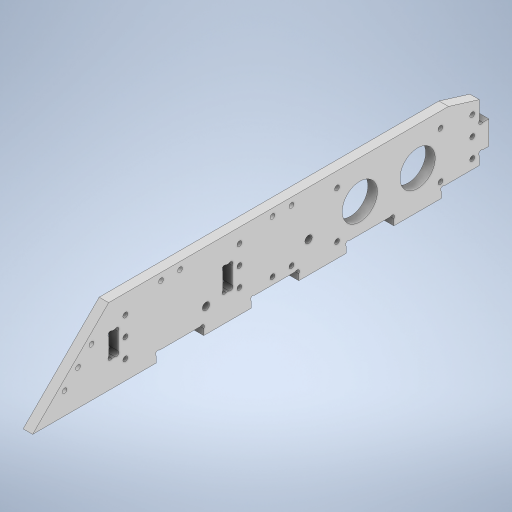
# Autodesk Inventor part: Inner Side Wall
Saved by Autodesk Inventor 2023 (Build 270158000, 158)
## iProperties
Created: 2022-12-26
Part Number: Inner Side Wall
Material: Generic
Document SubType Name: Modeling
Designer: justi
Density: 1 g/cm^3
Appearance: Default
Mass: 603.336 g
Surface Area: 1244.42 cm^2
Volume: 603.336 cm^3
Author: justi
Autodesk Inventor part; units mm, degrees
ref_plane "YZ Plane" through (0, 0, 0) normal (1, 0, 0) x (0, 1, 0)
ref_plane "XZ Plane" through (0, 0, 0) normal (0, 1, 0) x (-1, 0, 0)
ref_plane "XY Plane" through (0, 0, 0) normal (0, 0, 1) x (1, 0, 0)
sketch "Sketch1" plane through (0, 0, 0) normal (1, 0, 0) x (0, 1, 0)
  line L0 (0, 0) -> (101.6, 0)
  line L1 (101.6, 0) -> (101.6, -508)
  line L2 (101.6, -508) -> (0, -508)
  line L3 (0, -508) -> (0, 0)
  line L4 (0, 0) -> (0, 101.6)
  line L5 (0, 101.6) -> (101.6, 0)
  circle A0 centre (50.8, -412.75) radius 20.6375
  circle A1 centre (81.788, -443.23) radius 3.175
  circle A2 centre (19.812, -443.23) radius 3.175
  circle A3 centre (81.788, -305.054) radius 3.175
  circle A4 centre (19.812, -305.054) radius 3.175
  line L6 (66.675, 0) -> (34.925, 0)
  line L7 (34.925, 0) -> (34.925, -12.7)
  line L8 (34.925, -12.7) -> (66.675, -12.7)
  line L9 (66.675, -12.7) -> (66.675, 0)
  line L10 (66.675, -152.4) -> (34.925, -152.4)
  line L11 (34.925, -152.4) -> (34.925, -165.1)
  line L12 (34.925, -165.1) -> (66.675, -165.1)
  line L13 (66.675, -165.1) -> (66.675, -152.4)
  line L14 (0, -63.5) -> (12.7, -63.5)
  line L15 (12.7, -63.5) -> (12.7, -127)
  line L16 (12.7, -127) -> (0, -127)
  line L17 (0, -127) -> (0, -63.5)
  line L18 (0, -190.5) -> (12.7, -190.5)
  line L19 (12.7, -190.5) -> (12.7, -254)
  line L20 (12.7, -254) -> (0, -254)
  line L21 (0, -254) -> (0, -190.5)
  line L22 (0, -317.5) -> (12.7, -317.5)
  line L23 (12.7, -317.5) -> (12.7, -381)
  line L24 (12.7, -381) -> (0, -381)
  line L25 (0, -381) -> (0, -317.5)
  line L26 (0, -444.5) -> (12.7, -444.5)
  line L27 (12.7, -444.5) -> (12.7, -508)
  line L28 (12.7, -508) -> (0, -508)
  line L29 (0, -508) -> (0, -444.5)
  point P0 (0, -127)
  point P1 (0, -254)
  point P2 (0, -381)
  dimension "d0" = 508
  dimension "d1" = 101.6
  dimension "d2" = 101.6
  dimension "d3" = 41.275
  dimension "d4" = 50.8
  dimension "d5" = 95.25
  dimension "d6" = 6.35
  dimension "d7" = 30.48
  dimension "d8" = 30.988
  dimension "d9" = 6.35
  dimension "d10" = 30.48
  dimension "d11" = 30.988
  dimension "d12" = 6.35
  dimension "d13" = 107.696
  dimension "d14" = 6.35
  dimension "d15" = 107.696
  dimension "d16" = 30.988
  dimension "d17" = 30.988
  dimension "d18" = 31.75
  dimension "d19" = 12.7
  dimension "d20" = 34.925
  dimension "d21" = 31.75
  dimension "d22" = 34.925
  dimension "d23" = 139.7
  dimension "d24" = 12.7
  dimension "d25" = 12.7
  dimension "d26" = 63.5
  dimension "d27" = 63.5
  dimension "d28" = 12.7
  dimension "d29" = 63.5
  dimension "d30" = 63.5
  dimension "d31" = 12.7
  dimension "d32" = 63.5
  dimension "d33" = 63.5
  dimension "d34" = 12.7
  dimension "d35" = 63.5
  dimension "d36" = 63.5
  constraints: 60 end point, 14 parallel, 7 horizontal, 7 perpendicular, 5 centre point, 5 point on line, 1 vertical
  measures "d0" distance of L0.end L1.end
  measures "d1" distance of L1.end L2.end
  measures "d2" distance of L0.start L4.end
  measures "d3" diameter of A0
  measures "d4" distance from line of L1 A0.centre
  measures "d5" distance from line of L2 A0.centre
  measures "d6" diameter of A1
  measures "d7" vertical distance of A0.centre A1.centre
  measures "d8" horizontal distance of A0.centre A1.centre
  measures "d9" diameter of A2
  measures "d10" vertical distance of A0.centre A2.centre
  measures "d11" horizontal distance of A0.centre A2.centre
  measures "d12" diameter of A3
  measures "d13" vertical distance of A0.centre A3.centre
  measures "d14" diameter of A4
  measures "d15" vertical distance of A0.centre A4.centre
  measures "d16" horizontal distance of A4.centre A0.centre
  measures "d17" horizontal distance of A3.centre A0.centre
  measures "d18" distance of L8.end L7.end
  measures "d19" distance of L8.end L6.start
  measures "d20" distance between parallel lines of L1 L9
  measures "d21" distance of L12.end L11.end
  measures "d22" distance between parallel lines of L1 L13
  measures "d23" distance between parallel lines of L8 L10
  measures "d24" distance of L10.end L11.end
  measures "d25" distance of L15.end L16.end
  measures "d26" distance of L14.end L15.end
  measures "d27" distance between parallel lines of L0 L14
  measures "d28" distance of L19.end L20.end
  measures "d29" distance of L18.end L19.end
  measures "d30" distance between parallel lines of L16 L18
  measures "d31" distance of L23.end L24.end
  measures "d32" distance of L22.end L23.end
  measures "d33" distance between parallel lines of L20 L22
  measures "d34" distance of L27.end L28.end
  measures "d35" distance of L26.end L27.end
  measures "d36" distance between parallel lines of L24 L26
extrude "Extrusion1" add sketch "Sketch1" along normal blind 12.7 contours L4 L5 L0 | L0 L7 L8 L9 L1 L2 L27 L26 L3 L24 L23 L22 L20 L19 L18 L16 L15 L14
sketch "Sketch4" plane through (12.7, 0, 0) normal (1, 0, 0) x (0, 0, -1)
  line L0 (444.5, 12.7) -> (508, 12.7) projected
  line L1 (508, 12.7) -> (495.3, 12.7)
  line L2 (495.3, 12.7) -> (495.3, 28.575)
  line L3 (495.3, 28.575) -> (508, 28.575)
  line L4 (508, 28.575) -> (508, 12.7)
  line L5 (508, 101.6) -> (0, 101.6) projected
  line L6 (508, 101.6) -> (495.3, 101.6)
  line L7 (495.3, 101.6) -> (495.3, 60.325)
  line L8 (495.3, 60.325) -> (508, 60.325)
  line L9 (508, 60.325) -> (508, 101.6)
  circle A0 centre (412.75, 50.8) radius 20.6375 projected
  line L10 (412.75, 50.8) -> (400.05, 50.8)
  line L11 (400.05, 50.8) -> (400.05, 114.3)
  line L12 (400.05, 114.3) -> (412.75, 114.3)
  line L13 (412.75, 114.3) -> (412.75, 50.8)
  line L14 (412.75, 114.3) -> (495.3, 88.9)
  line L15 (495.3, 101.6) -> (495.3, 88.9)
  line L16 (495.3, 101.6) -> (454.025, 101.6)
  point P0 (0, 0)
  dimension "d39" = 12.7
  dimension "d40" = 15.875
  dimension "d41" = 12.7
  dimension "d42" = 31.75
  dimension "d43" = 12.7
  dimension "d44" = 63.5
  dimension "d45" = 12.7
  constraints: 30 end point, 6 parallel, 3 horizontal, 3 perpendicular, 2 point on line, 1 collinear, 1 midpoint
  measures "d39" distance of L2.end L3.end
  measures "d40" distance of L1.end L2.end
  measures "d41" distance of L8.end L7.end
  measures "d42" distance between parallel lines of L3 L8
  measures "d43" distance of L11.end L12.end
  measures "d44" distance of L12.end L10.start
  measures "d45" distance of L6.end L14.end
extrude "Extrusion2" cut sketch "Sketch4" against normal blind 12.7 contours L2 L3 L4 L0 | L9 L8 L7 L5 | L7 L14 L5
sketch "Sketch10" plane through (12.7, 0, 0) normal (1, 0, 0) x (0, 0, -1)
  line L0 (0, 66.675) -> (2.2451, 64.4299)
  line L1 (0, 66.675) -> (12.7, 66.675) projected
  line L2 (12.7, 66.675) -> (10.4549, 64.4299)
  line L3 (12.7, 66.675) -> (12.7, 34.925) projected
  line L4 (12.7, 34.925) -> (0, 34.925) projected
  line L5 (0, 34.925) -> (2.2451, 37.1701)
  line L6 (12.7, 34.925) -> (10.4549, 37.1701)
  line L7 (63.5, 12.7) -> (65.7451, 10.4549)
  line L8 (63.5, 12.7) -> (127, 12.7) projected
  line L9 (127, 12.7) -> (127, 0) projected
  line L10 (127, 12.7) -> (124.7549, 10.4549)
  line L11 (152.4, 34.925) -> (152.4, 66.675) projected
  line L12 (152.4, 66.675) -> (154.6451, 64.4299)
  line L13 (152.4, 66.675) -> (165.1, 66.675) projected
  line L14 (165.1, 66.675) -> (165.1, 34.925) projected
  line L15 (165.1, 66.675) -> (162.8549, 64.4299)
  line L16 (165.1, 34.925) -> (152.4, 34.925) projected
  line L17 (152.4, 34.925) -> (154.6451, 37.1701)
  line L18 (165.1, 34.925) -> (162.8549, 37.1701)
  line L19 (190.5, 0) -> (190.5, 12.7) projected
  line L20 (190.5, 12.7) -> (192.7451, 10.4549)
  line L21 (190.5, 12.7) -> (254, 12.7) projected
  line L22 (254, 12.7) -> (251.7549, 10.4549)
  line L23 (254, 12.7) -> (254, 0) projected
  line L24 (317.5, 0) -> (317.5, 12.7) projected
  line L25 (317.5, 12.7) -> (319.7451, 10.4549)
  line L26 (317.5, 12.7) -> (381, 12.7) projected
  line L27 (381, 12.7) -> (381, 0) projected
  line L28 (381, 12.7) -> (378.7549, 10.4549)
  line L29 (444.5, 0) -> (444.5, 12.7) projected
  line L30 (444.5, 12.7) -> (446.7451, 10.4549)
  line L31 (444.5, 12.7) -> (495.3, 12.7) projected
  line L32 (495.3, 12.7) -> (495.3, 28.575) projected
  line L33 (495.3, 28.575) -> (497.5451, 26.3299)
  line L34 (495.3, 28.575) -> (508, 28.575) projected
  line L35 (495.3, 60.325) -> (508, 60.325) projected
  line L36 (495.3, 60.325) -> (497.5451, 62.5701)
  circle A0 centre (497.5451, 62.5701) radius 3.175
  circle A1 centre (497.5451, 26.3299) radius 3.175
  circle A2 centre (446.7451, 10.4549) radius 3.175
  circle A3 centre (378.7549, 10.4549) radius 3.175
  circle A4 centre (319.7451, 10.4549) radius 3.175
  circle A5 centre (251.7549, 10.4549) radius 3.175
  circle A6 centre (192.7451, 10.4549) radius 3.175
  circle A7 centre (154.6451, 64.4299) radius 3.175
  circle A8 centre (162.8549, 64.4299) radius 3.175
  circle A9 centre (154.6451, 37.1701) radius 3.175
  circle A10 centre (162.8549, 37.1701) radius 3.175
  circle A11 centre (2.2451, 37.1701) radius 3.175
  circle A12 centre (10.4549, 37.1701) radius 3.175
  circle A13 centre (2.2451, 64.4299) radius 3.175
  circle A14 centre (10.4549, 64.4299) radius 3.175
  circle A15 centre (65.7451, 10.4549) radius 3.175
  circle A16 centre (124.7549, 10.4549) radius 3.175
  point P0 (0, 0)
  dimension "d53" = 3.175
  dimension "d54" = 45
  dimension "d55" = 3.175
  dimension "d56" = 45
  dimension "d57" = 3.175
  dimension "d58" = 45
  dimension "d59" = 3.175
  dimension "d60" = 45
  dimension "d61" = 3.175
  dimension "d62" = 45
  dimension "d63" = 3.175
  dimension "d64" = 45
  dimension "d65" = 3.175
  dimension "d66" = 45
  dimension "d67" = 3.175
  dimension "d68" = 45
  dimension "d69" = 3.175
  dimension "d70" = 45
  dimension "d71" = 3.175
  dimension "d72" = 45
  dimension "d73" = 3.175
  dimension "d74" = 45
  dimension "d75" = 3.175
  dimension "d76" = 45
  dimension "d77" = 3.175
  dimension "d78" = 45
  dimension "d79" = 3.175
  dimension "d80" = 45
  dimension "d81" = 3.175
  dimension "d82" = 45
  dimension "d83" = 3.175
  dimension "d84" = 45
  dimension "d85" = 3.175
  dimension "d86" = 45
  dimension "d87" = 6.35
  dimension "d88" = 6.35
  dimension "d89" = 6.35
  dimension "d90" = 6.35
  dimension "d91" = 6.35
  dimension "d92" = 6.35
  dimension "d93" = 6.35
  dimension "d94" = 6.35
  dimension "d95" = 6.35
  dimension "d96" = 6.35
  dimension "d97" = 6.35
  dimension "d98" = 6.35
  dimension "d99" = 6.35
  dimension "d100" = 6.35
  dimension "d101" = 6.35
  dimension "d102" = 6.35
  dimension "d103" = 6.35
  constraints: 34 end point, 17 centre point, 12 point on line
  measures "d53" distance of L0.start L0.end
  measures "d54" angle of L1 L0
  measures "d55" distance of L1.end L2.end
  measures "d56" angle of L3 L2
  measures "d57" distance of L4.end L5.end
  measures "d58" angle of L4 L5
  measures "d59" distance of L3.end L6.end
  measures "d60" angle of L3 L6
  measures "d61" distance of L7.start L7.end
  measures "d62" angle of L8 L7
  measures "d63" distance of L8.end L10.end
  measures "d64" angle of L9 L10
  measures "d65" distance of L11.end L12.end
  measures "d66" angle of L13 L12
  measures "d67" distance of L13.end L15.end
  measures "d68" angle of L14 L15
  measures "d69" distance of L11.start L17.end
  measures "d70" angle of L16 L17
  measures "d71" distance of L14.end L18.end
  measures "d72" angle of L14 L18
  measures "d73" distance of L19.end L20.end
  measures "d74" angle of L21 L20
  measures "d75" distance of L21.end L22.end
  measures "d76" angle of L23 L22
  measures "d77" distance of L24.end L25.end
  measures "d78" angle of L26 L25
  measures "d79" distance of L26.end L28.end
  measures "d80" angle of L27 L28
  measures "d81" distance of L29.end L30.end
  measures "d82" angle of L31 L30
  measures "d83" distance of L32.end L33.end
  measures "d84" angle of L34 L33
  measures "d85" distance of L35.start L36.end
  measures "d86" angle of L35 L36
  measures "d87" diameter of A0
  measures "d88" diameter of A1
  measures "d89" diameter of A2
  measures "d90" diameter of A3
  measures "d91" diameter of A4
  measures "d92" diameter of A5
  measures "d93" diameter of A6
  measures "d94" diameter of A7
  measures "d95" diameter of A8
  measures "d96" diameter of A9
  measures "d97" diameter of A10
  measures "d98" diameter of A11
  measures "d99" diameter of A12
  measures "d100" diameter of A13
  measures "d101" diameter of A14
  measures "d102" diameter of A15
  measures "d103" diameter of A16
extrude "Extrusion4" cut sketch "Sketch10" against normal blind 12.7 contours A13 L1 | L1 A13 | A14 L1 | L1 L3 A14 | A14 L3 | A12 L3 | L3 L4 A12 | A12 L4 | A11 L4 | L4 A11 | A15 L8 | L8 A15 | A16 L8 | L8 L9 A16 | A16 L9 | A9 L11 | L11 A9 L16 | L16 A9 | A7 L11 | L11 L13 A7 | A10 L14 L16 | L16 A10 | A7 L13 | L14 A10 | A8 L13 L14 | L14 A8 | A8 L13 | A6 L19 | L19 L21 A6 | A6 L21 | A5 L21 | L21 L23 A5 | A5 L23 | A4 L24 | L24 L26 A4 | A4 L26 | A3 L26 | L26 L27 A3 | A3 L27 | A2 L29 | L29 L31 A2 | A2 L31 | A1 L32 | L32 L34 A1 | A1 L34 | A0 L35 | L35 A0
sketch "Sketch11" plane through (12.7, 0, 0) normal (1, 0, 0) x (0, 0, -1)
  line L0 (297.942, 88.9) -> (450.342, 88.9)
  line L1 (450.342, 88.9) -> (450.342, 12.7)
  line L2 (450.342, 12.7) -> (297.942, 12.7)
  line L3 (297.942, 12.7) -> (297.942, 88.9)
  circle A0 centre (412.75, 50.8) radius 20.6375 projected
  circle A1 centre (443.23, 81.788) radius 3.175 projected
  circle A2 centre (174.625, 69.85) radius 3.175
  line L4 (165.1, 62.1849) -> (165.1, 39.4151) projected
  line L5 (454.025, 101.6) -> (0, 101.6) projected
  circle A3 centre (174.625, 44.45) radius 3.175
  line L6 (194.9901, 12.7) -> (249.5099, 12.7) projected
  circle A4 centre (22.225, 69.85) radius 3.175
  line L7 (12.7, 62.1849) -> (12.7, 39.4151) projected
  circle A5 centre (22.225, 44.45) radius 3.175
  line L8 (67.9901, 12.7) -> (122.5099, 12.7) projected
  circle A6 centre (485.775, 25.4) radius 3.175
  line L9 (448.9901, 12.7) -> (495.3, 12.7) projected
  line L10 (495.3, 12.7) -> (495.3, 24.0849) projected
  circle A7 centre (485.775, 50.8) radius 3.175
  line L11 (495.3, 64.8151) -> (495.3, 88.9) projected
  circle A8 centre (485.775, 76.2) radius 3.175
  circle A9 centre (244.221, 22.225) radius 3.175
  circle A10 centre (218.821, 22.225) radius 3.175
  circle A11 centre (-58.9438, 29.1858) radius 3.175
  circle A12 centre (-40.9833, 47.1463) radius 3.175
  line L12 (0, 101.6) -> (-101.6, 0) projected
  line L13 (-83.6395, 17.9605) -> (-29.758, 71.842)
  line L14 (-29.758, 71.842) -> (-16.2876, 58.3717)
  line L15 (-16.2876, 58.3717) -> (-70.1691, 4.4901)
  line L16 (-70.1691, 4.4901) -> (-83.6395, 17.9605)
  point P0 (0, 0)
  dimension "d106" = 152.4
  dimension "d107" = 76.2
  dimension "d108" = 38.1
  dimension "d109" = 7.112
  dimension "d110" = 6.35
  dimension "d111" = 9.525
  dimension "d112" = 31.75
  dimension "d113" = 6.35
  dimension "d114" = 9.525
  dimension "d115" = 31.75
  dimension "d116" = 6.35
  dimension "d117" = 31.75
  dimension "d118" = 9.525
  dimension "d119" = 6.35
  dimension "d120" = 9.525
  dimension "d121" = 31.75
  dimension "d122" = 6.35
  dimension "d123" = 12.7
  dimension "d124" = 9.525
  dimension "d125" = 6.35
  dimension "d126" = 9.525
  dimension "d127" = 25.4
  dimension "d128" = 6.35
  dimension "d129" = 9.525
  dimension "d130" = 25.4
  dimension "d131" = 6.35
  dimension "d132" = 9.525
  dimension "d133" = 6.35
  dimension "d134" = 9.525
  dimension "d135" = 25.4
  dimension "d136" = 53.721
  dimension "d139" = 6.35
  dimension "d140" = 6.35
  dimension "d141" = 19.05
  dimension "d142" = 76.2
  dimension "d143" = 25.4
  dimension "d144" = 9.525
  dimension "d145" = 9.525
  dimension "d146" = 25.4
  dimension "d147" = 25.4
  constraints: 16 end point, 11 centre point, 4 parallel, 2 perpendicular, 2 point on line, 1 horizontal
  measures "d106" distance of L1.end L2.end
  measures "d107" distance of L2.end L0.start
  measures "d108" distance from line of L0 A0.centre
  measures "d109" distance from line of L1 A1.centre
  measures "d110" diameter of A2
  measures "d111" distance from line of L4 A2.centre
  measures "d112" distance from line of L5 A2.centre
  measures "d113" diameter of A3
  measures "d114" distance from line of L4 A3.centre
  measures "d115" distance from line of L6 A3.centre
  measures "d116" diameter of A4
  measures "d117" distance from line of L5 A4.centre
  measures "d118" distance from line of L7 A4.centre
  measures "d119" diameter of A5
  measures "d120" distance from line of L7 A5.centre
  measures "d121" distance from line of L8 A5.centre
  measures "d122" diameter of A6
  measures "d123" distance from line of L9 A6.centre
  measures "d124" distance from line of L10 A6.centre
  measures "d125" diameter of A7
  measures "d126" distance from line of L11 A7.centre
  measures "d127" distance of A6.centre A7.centre
  measures "d128" diameter of A8
  measures "d129" distance from line of L11 A8.centre
  measures "d130" distance of A7.centre A8.centre
  measures "d131" diameter of A9
  measures "d132" distance from line of L6 A9.centre
  measures "d133" diameter of A10
  measures "d134" distance from line of L6 A10.centre
  measures "d135" distance of A9.centre A10.centre
  measures "d136" distance from line of L4 A10.centre
  measures "d139" diameter of A11
  measures "d140" diameter of A12
  measures "d141" distance of L13.end L14.end
  measures "d142" distance of L14.end L15.end
  measures "d143" distance from line of L12.end L16
  measures "d144" distance from line of L13 A11.centre
  measures "d145" distance from line of L13 A12.centre
  measures "d146" distance from line of L16 A11.centre
  measures "d147" distance of A12.centre A11.centre
extrude "Extrusion5" cut sketch "Sketch11" against normal blind 12.7 contours A2 | A3 | A4 | A5 | A6 | A7 | A8 | A9 | A10 | A11 | A12
sketch "Sketch19" plane through (12.7, 0, 0) normal (1, 0, 0) x (0, 0, -1)
  circle A0 centre (22.225, 57.15) radius 3.175
  line L0 (12.7, 62.1849) -> (12.7, 39.4151) projected
  circle A1 centre (22.225, 69.85) radius 3.175 projected
  circle A2 centre (22.225, 82.55) radius 3.175
  circle A3 centre (22.225, 31.75) radius 3.175
  point P0 (0, 0)
  dimension "d178" = 6.35
  dimension "d179" = 9.525
  dimension "d180" = 12.7
  dimension "d181" = 6.35
  dimension "d182" = 9.525
  dimension "d183" = 25.4
  dimension "d184" = 6.35
  dimension "d185" = 9.525
  dimension "d186" = 25.4
  constraints: 3 centre point
  measures "d178" diameter of A0
  measures "d179" distance from line of L0 A0.centre
  measures "d180" distance of A1.centre A0.centre
  measures "d181" diameter of A2
  measures "d182" distance from line of L0 A2.centre
  measures "d183" distance of A0.centre A2.centre
  measures "d184" diameter of A3
  measures "d185" distance from line of L0 A3.centre
  measures "d186" distance of A0.centre A3.centre
extrude "Extrusion8" cut sketch "Sketch19" against normal blind 12.7 contours A0 | A2 | A3
sketch "Sketch20" plane through (12.7, 0, 0) normal (1, 0, 0) x (0, 0, -1)
  circle A0 centre (22.225, 69.85) radius 3.175 projected
  circle A1 centre (22.225, 69.85) radius 3.175
  circle A2 centre (22.225, 44.45) radius 3.175 projected
  circle A3 centre (22.225, 44.45) radius 3.175
  point P0 (0, 0)
  dimension "d189" = 6.35
  dimension "d190" = 6.35
  constraints: 2 centre point, 2 coincident
  measures "d189" diameter of A1
  measures "d190" diameter of A3
extrude "Extrusion9" add sketch "Sketch20" against normal blind 12.7
sketch "Sketch22" plane through (12.7, 0, 0) normal (1, 0, 0) x (0, 0, -1)
  circle A0 centre (412.75, 50.8) radius 20.6375 projected
  circle A1 centre (412.75, 50.8) radius 23.495
  circle A2 centre (335.534, 50.8) radius 23.495
  circle A3 centre (305.054, 81.788) radius 3.175 projected
  point P0 (0, 0)
  dimension "d198" = 46.99
  dimension "d199" = 46.99
  dimension "d200" = 77.216
  dimension "d201" = 30.988
  constraints: 2 centre point, 1 coincident
  measures "d198" diameter of A1
  measures "d199" diameter of A2
  measures "d200" distance of A1.centre A2.centre
  measures "d201" vertical distance of A3.centre A2.centre
extrude "Extrusion10" cut sketch "Sketch22" against normal blind 12.7 contours A1 | A2
sketch "Sketch23" plane through (12.7, 0, 0) normal (1, 0, 0) x (0, 0, -1)
  circle A0 centre (218.821, 92.075) radius 3.175
  line L0 (454.025, 101.6) -> (0, 101.6) projected
  line L1 (165.1, 62.1849) -> (165.1, 39.4151) projected
  circle A1 centre (244.221, 92.075) radius 3.175
  point P0 (0, 0)
  dimension "d204" = 6.35
  dimension "d205" = 9.525
  dimension "d206" = 53.721
  dimension "d207" = 6.35
  dimension "d208" = 9.525
  dimension "d209" = 25.4
  constraints: 2 centre point
  measures "d204" diameter of A0
  measures "d205" distance from line of L0 A0.centre
  measures "d206" distance from line of L1 A0.centre
  measures "d207" diameter of A1
  measures "d208" distance from line of L0 A1.centre
  measures "d209" distance of A0.centre A1.centre
extrude "Extrusion11" cut sketch "Sketch23" against normal blind 12.7
sketch "Sketch24" plane through (12.7, 0, 0) normal (1, 0, 0) x (0, 0, -1)
  circle A0 centre (174.625, 57.15) radius 3.175
  circle A1 centre (174.625, 82.55) radius 3.175
  circle A2 centre (174.625, 31.75) radius 3.175
  line L0 (165.1, 62.1849) -> (165.1, 39.4151) projected
  line L1 (454.025, 101.6) -> (0, 101.6) projected
  point P0 (0, 0)
  dimension "d212" = 6.35
  dimension "d213" = 6.35
  dimension "d214" = 6.35
  dimension "d215" = 9.525
  dimension "d216" = 44.45
  dimension "d217" = 25.4
  dimension "d218" = 25.4
  constraints: 3 centre point
  measures "d212" diameter of A0
  measures "d213" diameter of A1
  measures "d214" diameter of A2
  measures "d215" distance from line of L0 A0.centre
  measures "d216" distance from line of L1 A0.centre
  measures "d217" distance of A1.centre A0.centre
  measures "d218" distance of A0.centre A2.centre
extrude "Extrusion12" cut sketch "Sketch24" against normal blind 12.7
sketch "Sketch25" plane through (12.7, 0, 0) normal (1, 0, 0) x (0, 0, -1)
  circle A0 centre (174.625, 69.85) radius 3.175 projected
  circle A1 centre (174.625, 69.85) radius 3.175
  circle A2 centre (174.625, 44.45) radius 3.175 projected
  circle A3 centre (174.625, 44.45) radius 3.175
  point P0 (0, 0)
  dimension "d221" = 6.35
  dimension "d222" = 6.35
  constraints: 2 centre point, 2 coincident
  measures "d221" diameter of A1
  measures "d222" diameter of A3
extrude "Extrusion13" add sketch "Sketch25" against normal blind 12.7
sketch "Sketch28" plane through (12.7, 0, 0) normal (1, 0, 0) x (0, 0, -1)
  circle A0 centre (69.85, 92.075) radius 3.175
  circle A1 centre (95.25, 92.075) radius 3.175
  line L0 (454.025, 101.6) -> (0, 101.6) projected
  line L1 (12.7, 62.1849) -> (12.7, 39.4151) projected
  point P0 (0, 0)
  dimension "d225" = 6.35
  dimension "d226" = 6.35
  dimension "d227" = 9.525
  dimension "d228" = 9.525
  dimension "d229" = 25.4
  dimension "d230" = 57.15
  constraints: 2 centre point
  measures "d225" diameter of A0
  measures "d226" diameter of A1
  measures "d227" distance from line of L0 A0.centre
  measures "d228" distance from line of L0 A1.centre
  measures "d229" distance of A0.centre A1.centre
  measures "d230" distance from line of L1 A0.centre
extrude "Extrusion14" cut sketch "Sketch28" against normal blind 12.7
sketch "Sketch33" plane through (12.7, 0, 0) normal (1, 0, 0) x (0, 0, -1)
  circle A0 centre (22.225, 31.75) radius 3.175 projected
  circle A1 centre (22.225, 31.75) radius 3.175
  circle A2 centre (22.225, 57.15) radius 3.175 projected
  circle A3 centre (22.225, 57.15) radius 3.175
  circle A4 centre (22.225, 82.55) radius 3.175 projected
  circle A5 centre (22.225, 82.55) radius 3.175
  point P0 (0, 0)
  constraints: 3 centre point, 3 coincident
extrude "Extrusion16" add sketch "Sketch33" against normal blind 12.7
sketch "Sketch34" plane through (12.7, 0, 0) normal (1, 0, 0) x (0, 0, -1)
  circle A0 centre (22.225, 25.4) radius 3.175
  line L0 (12.7, 62.1849) -> (12.7, 39.4151) projected
  line L1 (-101.6, 0) -> (63.5, 0) projected
  circle A1 centre (22.225, 50.8) radius 3.175
  circle A2 centre (22.225, 76.2) radius 3.175
  circle A3 centre (412.75, 50.8) radius 23.495 projected
  circle A4 centre (412.75, 50.8) radius 76.2
  circle A5 centre (22.225, 25.4) radius 38.1
  line L2 (412.75, -25.4) -> (20.9886, -12.6799)
  line L3 (20.9886, -12.6799) -> (-119.6611, -8.1132)
  line L4 (-101.6, 0) -> (63.5, 0) projected
  line L5 (-101.6, 0) -> (-101.6, -6.2484)
  line L6 (22.225, 25.4) -> (412.75, 50.8)
  circle A6 centre (129.9474, 32.4063) radius 4.7625
  circle A7 centre (267.0079, 41.3208) radius 4.7625
  point P0 (0, 0)
  dimension "d250" = 152.4
  dimension "d251" = 76.2
  dimension "d242" = 6.35
  dimension "d243" = 9.525
  dimension "d244" = 25.4
  dimension "d245" = 6.35
  dimension "d246" = 9.525
  dimension "d247" = 25.4
  dimension "d248" = 6.35
  dimension "d249" = 25.4
  dimension "d252" = 6.2484
  dimension "d253" = 9.525
  dimension "d254" = 107.95
  dimension "d255" = 9.525
  dimension "d256" = 146.05
  constraints: 8 end point, 5 centre point, 3 point on line, 2 coincident, 1 vertical, 1 vertical alignment, 7 other
  measures "d242" diameter of A0
  measures "d243" distance from line of L0 A0.centre
  measures "d244" distance from line of L1 A0.centre
  measures "d245" diameter of A1
  measures "d246" distance from line of L0 A1.centre
  measures "d247" distance of A0.centre A1.centre
  measures "d248" diameter of A2
  measures "d249" distance of A1.centre A2.centre
  measures "d252" distance of L1.start L5.end
  measures "d253" diameter of A6
  measures "d254" distance of A0.centre A6.centre
  measures "d255" diameter of A7
  measures "d256" distance of point (412.75, 50.8) A7.centre
extrude "Extrusion17" cut sketch "Sketch34" against normal blind 12.7 contours A0 | A6 L6 | L6 A6 | A7 L6 | L6 A7 | A1 | A2
sketch "Sketch37" plane through (12.7, 0, 0) normal (1, 0, 0) x (0, 0, -1)
  circle A0 centre (-23.0228, 65.1069) radius 3.175
  line L0 (0, 101.6) -> (-101.6, 0) projected
  circle A1 centre (-40.9833, 47.1463) radius 3.175 projected
  line L1 (-20.7777, 80.8223) -> (-74.6592, 26.9408)
  line L2 (-74.6592, 26.9408) -> (-61.1888, 13.4704)
  line L3 (-61.1888, 13.4704) -> (-7.3073, 67.3519)
  line L4 (-7.3073, 67.3519) -> (-20.7777, 80.8223)
  circle A2 centre (-58.9438, 29.1858) radius 3.175 projected
  point P0 (0, 0)
  dimension "d263" = 6.35
  dimension "d264" = 9.525
  dimension "d265" = 25.4
  dimension "d266" = 19.05
  dimension "d267" = 76.2
  dimension "d268" = 12.7
  constraints: 8 end point, 2 parallel, 2 point on line, 1 centre point, 1 perpendicular
  measures "d263" diameter of A0
  measures "d264" distance from line of L0 A0.centre
  measures "d265" distance of A1.centre A0.centre
  measures "d266" distance of L2.end L1.end
  measures "d267" distance of L2.end L3.end
  measures "d268" distance from line of L2 A2.centre
extrude "Extrusion18" cut sketch "Sketch37" against normal blind 12.7 contours A0
body "Solid1"
